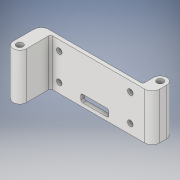
# Autodesk Inventor part: US Halterung rechts
Saved by Autodesk Inventor 2018 (Build 220112000, 112)
## iProperties
Created: 2019-03-05
Part Number: US Halterung rechts
Material: ABS-Kunststoff
Document SubType Name: Modeling
Designer: RedBots
Density: 0.767693 g/cm^3
Appearance: Glatt - weiß
Mass: 5 g
Surface Area: 52.6611 cm^2
Volume: 6.51302 cm^3
Author: RedBots
Autodesk Inventor part; units mm, degrees
ref_plane "YZ Plane" through (0, 0, 0) normal (1, 0, 0) x (0, 1, 0)
ref_plane "XZ Plane" through (0, 0, 0) normal (0, 1, 0) x (-1, 0, 0)
ref_plane "XY Plane" through (0, 0, 0) normal (0, 0, 1) x (1, 0, 0)
sketch "Skizze2" plane through (0, 0, 0) normal (0, 0, 1) x (1, 0, 0)
  line L0 (0, 0) -> (36.75, -63.6529) construction
  line L1 (0, 0) -> (73.5, 0) construction
  line L2 (36.75, -63.6529) -> (20.2955, -73.1529) construction
  line L3 (0, 0) -> (-34.202, -93.9693) construction
  line L4 (0, 0) -> (100, 0) construction
  circle A0 centre (-34.202, -93.9693) radius 1.75
  circle A1 centre (20.2955, -73.1529) radius 1.75
  arc A2 (-37.702, -93.9693) -> (-30.702, -93.9693) centre (-34.202, -93.9693) ccw
  arc A3 (23.7955, -73.1529) -> (16.7955, -73.1529) centre (20.2955, -73.1529) ccw
  line L5 (-37.702, -93.9693) -> (-37.702, -78.9693)
  line L6 (-37.702, -78.9693) -> (16.7955, -78.9693)
  line L7 (16.7955, -78.9693) -> (16.7955, -73.1529)
  line L8 (23.7955, -73.1529) -> (23.7955, -80.9693)
  line L9 (23.7955, -80.9693) -> (-30.702, -80.9693)
  line L10 (-30.702, -80.9693) -> (-30.702, -93.9693)
  line L11 (-30.702, -93.9693) -> (-37.702, -93.9693) construction
  line L12 (16.7955, -73.1529) -> (23.7955, -73.1529) construction
  dimension "d16" = 73.5
  dimension "d17" = 60
  dimension "d18" = 19
  dimension "d19" = 100
  dimension "d20" = 110
  dimension "d21" = 3.5
  dimension "d22" = 7
  dimension "d23" = 2
  dimension "d24" = 13
  constraints: 26 end point, 5 horizontal, 4 centre point, 4 coincident, 4 point on circle, 4 tangent, 3 equal length, 3 vertical, 2 perpendicular, 1 equal radius, 1 parallel
  measures "d16" distance of L0.start L0.end
  measures "d17" angle of L0 L1
  measures "d18" distance of L0.end L2.end
  measures "d19" distance of L0.start L3.end
  measures "d20" angle of L3 L4
  measures "d21" diameter of A0
  measures "d22" distance of L7.end L8.start
  measures "d23" distance between parallel lines of L9 L6
  measures "d24" distance from line of L9 L3.end
extrude "Extrusion2" add sketch "Skizze2" along normal blind 25
sketch "Skizze3" plane through (-30.702, -80.9693, 0) normal (0, -1, 0) x (1, 0, 0)
  line L0 (4.6988, 19.739) -> (42.7988, 19.739) construction
  line L1 (42.7988, 19.739) -> (42.7988, 5.261) construction
  line L2 (42.7988, 5.261) -> (4.6988, 5.261) construction
  line L3 (4.6988, 5.261) -> (4.6988, 19.739) construction
  line L4 (0, 0) -> (0, 25) construction
  line L5 (0, 12.5) -> (47.4975, 12.5) construction
  line L6 (47.4975, 0) -> (47.4975, 25) construction
  line L7 (0, 25) -> (54.4975, 25) construction
  line L8 (23.7488, 25) -> (23.7488, 0) construction
  line L9 (0, 0) -> (54.4975, 0) construction
  circle A0 centre (42.7988, 19.739) radius 1.5
  circle A1 centre (4.6988, 5.261) radius 1.5
  line L10 (2.1588, 22.4949) -> (45.3388, 22.4949) construction
  line L11 (45.3388, 22.4949) -> (45.3388, 2.5051) construction
  line L12 (45.3388, 2.5051) -> (2.1588, 2.5051) construction
  line L13 (2.1588, 2.5051) -> (2.1588, 22.4949) construction
  line L14 (16.2488, 2.0051) -> (31.2488, 2.0051)
  line L15 (31.2488, 2.0051) -> (31.2488, 6.0051)
  line L16 (31.2488, 6.0051) -> (16.2488, 6.0051)
  line L17 (16.2488, 6.0051) -> (16.2488, 2.0051)
  circle A2 centre (4.6988, 19.739) radius 1.5
  circle A3 centre (42.7988, 5.261) radius 1.5
  point P0 (30.702, 0)
  point P1 (23.7488, 12.5)
  point P2 (23.7488, 19.739)
  point P3 (42.7988, 12.5)
  point P4 (23.7488, 22.4949)
  point P5 (45.3388, 12.5)
  point P6 (23.7488, 6.0051)
  dimension "d27" = 38.1
  dimension "d28" = 14.478
  dimension "d29" = 3
  dimension "d30" = 43.18
  dimension "d31" = 19.9898
  dimension "d32" = 15
  dimension "d33" = 4
  dimension "d39" = 0.5
  constraints: 28 end point, 9 midpoint, 7 point on line, 6 parallel, 4 centre point, 4 coincident, 3 equal radius, 3 horizontal, 3 perpendicular, 1 vertical
  measures "d27" distance of L0.start L0.end
  measures "d28" distance of L0.end L1.end
  measures "d29" diameter of A0
  measures "d30" distance of L10.start L10.end
  measures "d31" distance of L10.end L11.end
  measures "d32" distance of L16.end L15.end
  measures "d33" distance of L15.end L14.end
  measures "d39" distance between parallel lines of L12 L14
extrude "Extrusion3" cut sketch "Skizze3" against normal up to next
fillet "Rundung1" radius 1 4 edges at (-14.4532, -79.9693, 2.0051) (-14.4532, -79.9693, 6.0051) (0.5468, -79.9693, 2.0051) (0.5468, -79.9693, 6.0051)
fillet "Rundung2" radius 4 2 edges at (23.7955, -80.9693, 12.5) (-37.702, -78.9693, 12.5)
fillet "Rundung3" radius 1 2 edges at (16.7955, -78.9693, 12.5) (-30.702, -80.9693, 12.5)
